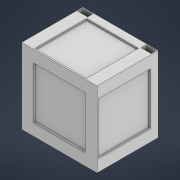
# Autodesk Inventor part: Joint_MarkerCube_V3
Saved by Autodesk Inventor 2022 (Build 260153000, 153)
## iProperties
Created: 2023-05-10
Part Number: Joint_MarkerCube_V3
Material: Generic
Document SubType Name: Modeling
Designer: Karl Spiteri
Density: 1 g/cm^3
Appearance: Default
Author: Karl Spiteri
Autodesk Inventor part; units mm, degrees
ref_plane "YZ Plane" through (0, 0, 0) normal (1, 0, 0) x (0, 1, 0)
ref_plane "XZ Plane" through (0, 0, 0) normal (0, 1, 0) x (-1, 0, 0)
ref_plane "XY Plane" through (0, 0, 0) normal (0, 0, 1) x (1, 0, 0)
sketch "Sketch7" plane through (0, 0, 0) normal (0, 0, 1) x (1, 0, 0)
  line L0 (0, 0) -> (-80, 0)
  line L1 (-80, 0) -> (-80, 80)
  line L2 (-80, 80) -> (0, 80)
  line L3 (0, 80) -> (0, 0)
  line L4 (-70, 10) -> (-10, 10)
  line L5 (-10, 10) -> (-10, 70)
  line L6 (-10, 70) -> (-70, 70)
  line L7 (-70, 70) -> (-70, 10)
  dimension "d54" = 80
  dimension "d55" = 80
  dimension "d110" = 60
  dimension "d111" = 60
  constraints: 16 end point, 4 parallel, 2 horizontal, 2 perpendicular
  measures "d54" distance of L1.end L2.end
  measures "d55" distance of L0.end L1.end
  measures "d110" distance of L6.end L5.end
  measures "d111" distance of L5.end L4.end
extrude "Extrusion10" add sketch "Sketch7" along normal blind 60 contours L0 L1 L2 L3 | L7 L6 L5 L4
sketch "Sketch8" plane through (0, 0, 60) normal (0, 0, 1) x (1, 0, 0)
  line L0 (0, 0) -> (0, 80) projected
  line L1 (0, 0) -> (-80, 0)
  line L2 (-80, 0) -> (-80, 80)
  line L3 (-80, 80) -> (0, 80)
  line L4 (0, 80) -> (0, 0)
  dimension "d60" = 80
  dimension "d61" = 80
  constraints: 8 end point, 2 parallel, 1 horizontal, 1 perpendicular
  measures "d60" distance of L2.end L3.end
  measures "d61" distance of L1.end L2.end
extrude "Extrusion11" add sketch "Sketch8" along normal blind 5
sketch "Sketch9" plane through (0, 0, 65) normal (0, 0, 1) x (1, 0, 0)
  line L0 (-12.5, 12.5) -> (-67.5, 12.5)
  line L1 (-67.5, 12.5) -> (-67.5, 67.5)
  line L2 (-67.5, 67.5) -> (-12.5, 67.5)
  line L3 (-12.5, 67.5) -> (-12.5, 12.5)
  point P0 (0, 0)
  dimension "d64" = 55
  dimension "d65" = 55
  constraints: 8 end point, 2 parallel, 1 horizontal, 1 perpendicular
  measures "d64" distance of L1.end L2.end
  measures "d65" distance of L0.end L1.end
extrude "Extrusion12" cut sketch "Sketch9" against normal blind 2
sketch "Sketch10" plane through (0, 0, 0) normal (1, 0, 0) x (0, 0, -1)
  line L0 (-63.5, 12.5) -> (-8.5, 12.5)
  line L1 (-8.5, 12.5) -> (-8.5, 67.5)
  line L2 (-8.5, 67.5) -> (-63.5, 67.5)
  line L3 (-63.5, 67.5) -> (-63.5, 12.5)
  point P0 (0, 0)
  dimension "d68" = 55
  dimension "d69" = 55
  constraints: 8 end point, 2 parallel, 1 horizontal, 1 perpendicular
  measures "d68" distance of L2.end L1.end
  measures "d69" distance of L1.end L0.end
extrude "Extrusion13" cut sketch "Sketch10" against normal blind 2
sketch "Sketch11" plane through (-80, 80, 0) normal (0, 1, 0) x (1, 0, 0)
  line L0 (12.5, -63.5) -> (67.5, -63.5)
  line L1 (67.5, -63.5) -> (67.5, -8.5)
  line L2 (67.5, -8.5) -> (12.5, -8.5)
  line L3 (12.5, -8.5) -> (12.5, -63.5)
  point P0 (80, 0)
  dimension "d72" = 55
  dimension "d73" = 55
  constraints: 8 end point, 2 parallel, 1 horizontal, 1 perpendicular
  measures "d72" distance of L2.end L1.end
  measures "d73" distance of L1.end L0.end
sketch "Sketch12" plane through (-80, 0, 0) normal (-1, 0, 0) x (0, 0, 1)
  line L0 (63.5, 12.5) -> (8.5, 12.5)
  line L1 (8.5, 12.5) -> (8.5, 67.5)
  line L2 (8.5, 67.5) -> (63.5, 67.5)
  line L3 (63.5, 67.5) -> (63.5, 12.5)
  point P0 (0, 0)
  dimension "d74" = 55
  dimension "d75" = 55
  constraints: 8 end point, 2 parallel, 1 horizontal, 1 perpendicular
  measures "d74" distance of L1.end L2.end
  measures "d75" distance of L0.end L1.end
sketch "Sketch13" plane through (-80, 0, 0) normal (0, -1, 0) x (1, 0, 0)
  line L0 (12.5, 63.5) -> (67.5, 63.5)
  line L1 (67.5, 63.5) -> (67.5, 8.5)
  line L2 (67.5, 8.5) -> (12.5, 8.5)
  line L3 (12.5, 8.5) -> (12.5, 63.5)
  point P0 (80, 0)
  dimension "d76" = 55
  dimension "d77" = 55
  constraints: 8 end point, 2 parallel, 1 horizontal, 1 perpendicular
  measures "d76" distance of L1.end L2.end
  measures "d77" distance of L0.end L1.end
extrude "Extrusion14" cut sketch "Sketch11" against normal blind 2
extrude "Extrusion15" cut sketch "Sketch12" against normal blind 2
extrude "Extrusion16" cut sketch "Sketch13" against normal blind 2
sketch "Sketch14" plane through (-80, 80, 0) normal (0, 1, 0) x (1, 0, 0)
  line L0 (79, -1) -> (68.4, -1)
  line L1 (68.4, -1) -> (68.4, -6.6)
  line L2 (68.4, -6.6) -> (79, -6.6)
  line L3 (79, -6.6) -> (79, -1)
  line L4 (1, -1) -> (11.6, -1)
  line L5 (11.6, -1) -> (11.6, -6.6)
  line L6 (11.6, -6.6) -> (1, -6.6)
  line L7 (1, -6.6) -> (1, -1)
  point P0 (80, 0)
  dimension "d84" = 10.6
  dimension "d85" = 5.6
  dimension "d86" = 10.6
  dimension "d87" = 5.6
  constraints: 16 end point, 4 parallel, 2 horizontal, 2 perpendicular
  measures "d84" distance of L2.end L1.end
  measures "d85" distance of L1.end L0.end
  measures "d86" distance of L5.end L6.end
  measures "d87" distance of L4.end L5.end
extrude "Extrusion17" cut sketch "Sketch14" against normal blind 5
sketch "Sketch16" plane through (-80, 0, 0) normal (0, -1, 0) x (1, 0, 0)
  line L0 (1, 1) -> (11.6, 1)
  line L1 (11.6, 1) -> (11.6, 6.6)
  line L2 (11.6, 6.6) -> (1, 6.6)
  line L3 (1, 6.6) -> (1, 1)
  line L4 (79, 1) -> (68.4, 1)
  line L5 (68.4, 1) -> (68.4, 6.6)
  line L6 (68.4, 6.6) -> (79, 6.6)
  line L7 (79, 6.6) -> (79, 1)
  point P0 (80, 0)
  dimension "d94" = 10.6
  dimension "d95" = 5.6
  dimension "d96" = 10.6
  dimension "d97" = 5.6
  constraints: 16 end point, 4 parallel, 2 horizontal, 2 perpendicular
  measures "d94" distance of L2.end L1.end
  measures "d95" distance of L1.end L0.end
  measures "d96" distance of L5.end L6.end
  measures "d97" distance of L4.end L5.end
extrude "Extrusion19" cut sketch "Sketch16" against normal blind 5
sketch "Sketch18" plane through (0, 0, 0) normal (0, 0, -1) x (-1, 0, 0)
  line L0 (10, 10) -> (70, 10)
  line L1 (70, 10) -> (70, 70)
  line L2 (70, 70) -> (10, 70)
  line L3 (10, 70) -> (10, 10)
  point P0 (0, 0)
  dimension "d114" = 60
  dimension "d115" = 60
  constraints: 8 end point, 2 parallel, 1 horizontal, 1 perpendicular
  measures "d114" distance of L2.end L1.end
  measures "d115" distance of L1.end L0.end
extrude "Extrusion21" cut sketch "Sketch18" against normal blind 60
body "Solid6"
